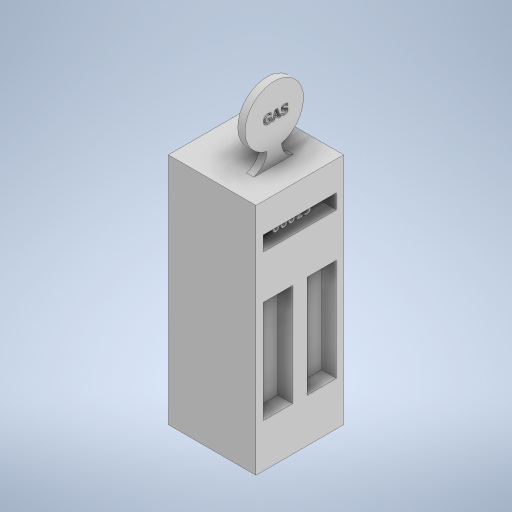
# Autodesk Inventor part: gaspomp
Saved by Autodesk Inventor 2023 (Build 270158000, 158)
## iProperties
Created: 2023-06-06
Part Number: gaspomp
Material: Generic
Document SubType Name: Modeling
Designer: Prestige
Density: 1 g/cm^3
Appearance: Default
Author: Prestige
Autodesk Inventor part; units mm, degrees
ref_plane "YZ Plane" through (0, 0, 0) normal (1, 0, 0) x (0, 1, 0)
ref_plane "XZ Plane" through (0, 0, 0) normal (0, 1, 0) x (-1, 0, 0)
ref_plane "XY Plane" through (0, 0, 0) normal (0, 0, 1) x (1, 0, 0)
sketch "Sketch1" plane through (0, 0, 0) normal (0, 1, 0) x (-1, 0, 0)
  line L0 (0, 0) -> (10, 0)
  line L1 (10, 0) -> (10, -10)
  line L2 (10, -10) -> (0, -10)
  line L3 (0, -10) -> (0, 0)
  dimension "d0" = 10
  dimension "d1" = 10
  constraints: 8 end point, 2 parallel, 1 horizontal, 1 perpendicular
  measures "d0" distance of L0.end L1.end
  measures "d1" distance of L1.end L2.end
extrude "Extrusion1" add sketch "Sketch1" along normal blind 5
sketch "Sketch2" plane through (0, 5, 0) normal (0, 1, 0) x (1, 0, 0)
  line L0 (10, -10) -> (-20, -10)
  line L1 (-20, -10) -> (-20, 20)
  line L2 (-20, 20) -> (10, 20)
  line L3 (10, 20) -> (10, -10)
  line L4 (0, 10) -> (-10, 10) projected
  line L5 (-10, 10) -> (-10, 0) projected
  point P0 (0, 0)
  point P1 (-5, 10)
  point P2 (-10, 5)
  dimension "d4" = 30
  dimension "d5" = 30
  dimension "d6" = 10
  dimension "d7" = 10
  constraints: 8 end point, 2 midpoint, 2 parallel, 1 horizontal, 1 perpendicular
  measures "d4" distance of L0.end L1.end
  measures "d5" distance of L1.end L2.end
  measures "d6" distance from line of point (-5, 10) L2
  measures "d7" distance from line of L1 point (-10, 5)
extrude "Extrusion2" add sketch "Sketch2" along normal blind 80
sketch "Sketch3" plane through (0, 0, 0) normal (1, 0, 0) x (0, 1, 0)
  arc A0 (90.3175, -7.5) -> (90.3175, -2.5) centre (100, -5) ccw
  line L0 (85, 10) -> (85, -20) projected
  line L1 (85, -20) -> (85, 10) projected
  line L2 (85, -2.5) -> (85, -7.5)
  line L3 (5, 10) -> (85, 10) projected
  arc A1 (90.3175, -7.5) -> (85, -14.4535) centre (90.3175, -13.01) ccw
  arc A2 (85, 5) -> (90.3175, -2.5) centre (90.8491, 3.5119) ccw
  point P0 (0, 0)
  point P1 (87.6588, -2.5)
  point P2 (85, 2.0239)
  point P3 (85, -11.5665)
  dimension "d10" = 20
  dimension "d11" = 15
  dimension "d13" = 2.5
  dimension "d14" = 15
  constraints: 6 point on circle, 3 centre point, 3 point on line, 2 end point
  measures "d10" diameter of A0
  measures "d11" distance from line of L0 A0.centre
  measures "d13" vertical distance of A0.centre point (87.659, -2.5)
  measures "d14" distance from line of L3 A0.centre
extrude "Extrusion3" add sketch "Sketch3" along normal mid plane 2.5 contours A1 L0 A2 A0
sketch "Sketch4" plane through (1.25, 0, 0) normal (1, 0, 0) x (0, 0, -1)
  line L0 (1.1377, 101.4111) -> (14.2751, 101.4111) construction
  line L1 (14.2751, 101.4111) -> (14.2751, 95.9848) construction
  line L2 (14.2751, 95.9848) -> (1.1377, 95.9848) construction
  line L3 (1.1377, 95.9848) -> (1.1377, 101.4111) construction
  spline S0 degree 2 poles (3.9999, 98.4748) (3.7997, 98.3933) (3.1595, 98.2376) (2.8481, 98.2376) knots 0 0 0 1 2 2 2
  spline S1 degree 2 poles (2.8481, 98.2376) (2.1289, 98.2376) (1.2761, 99.068) (1.2761, 99.8293) knots 0 0 0 1 2 2 2
  spline S2 degree 2 poles (1.2761, 99.8293) (1.2761, 100.5461) (2.1289, 101.4111) (2.8703, 101.4111) knots 0 0 0 1 2 2 2
  spline S3 degree 2 poles (2.8703, 101.4111) (3.2535, 101.4111) (3.7329, 101.2653) (3.9875, 101.1417) knots 0 0 0 1 2 2 2
  line L4 (3.9875, 101.1417) -> (3.9875, 100.425)
  line L5 (3.9875, 100.425) -> (3.9183, 100.425)
  spline S4 degree 2 poles (3.9183, 100.425) (3.8639, 100.467) (3.6563, 100.6276) (3.5575, 100.682) knots 0 0 0 1 2 2 2
  spline S5 degree 2 poles (3.5575, 100.682) (3.4438, 100.7487) (3.1422, 100.8427) (2.9742, 100.8427) knots 0 0 0 1 2 2 2
  spline S6 degree 2 poles (2.9742, 100.8427) (2.7789, 100.8427) (2.4551, 100.7191) (2.3291, 100.593) knots 0 0 0 1 2 2 2
  spline S7 degree 2 poles (2.3291, 100.593) (2.2079, 100.4694) (2.0671, 100.0913) (2.0671, 99.8416) knots 0 0 0 1 2 2 2
  spline S8 degree 2 poles (2.0671, 99.8416) (2.0671, 99.3078) (2.6034, 98.7986) (3.0656, 98.7986) knots 0 0 0 1 2 2 2
  spline S9 degree 2 poles (3.0656, 98.7986) (3.1076, 98.7986) (3.2164, 98.8036) (3.2584, 98.806) knots 0 0 0 1 2 2 2
  line L6 (3.2584, 98.806) -> (3.2584, 99.4066)
  line L7 (3.2584, 99.4066) -> (2.6677, 99.4066)
  line L8 (2.6677, 99.4066) -> (2.6677, 99.9776)
  line L9 (2.6677, 99.9776) -> (3.9999, 99.9776)
  line L10 (3.9999, 99.9776) -> (3.9999, 98.4748)
  line L11 (4.2495, 98.3018) -> (5.2802, 101.3518)
  line L12 (5.2802, 101.3518) -> (6.1156, 101.3518)
  line L13 (6.1156, 101.3518) -> (7.1463, 98.3018)
  line L14 (7.1463, 98.3018) -> (6.3578, 98.3018)
  line L15 (6.3578, 98.3018) -> (6.1675, 98.9247)
  line L16 (6.1675, 98.9247) -> (5.2085, 98.9247)
  line L17 (5.2085, 98.9247) -> (5.0157, 98.3018)
  line L18 (5.0157, 98.3018) -> (4.2495, 98.3018)
  line L19 (5.9994, 99.4783) -> (5.688, 100.4867)
  line L20 (5.688, 100.4867) -> (5.3741, 99.4783)
  line L21 (5.3741, 99.4783) -> (5.9994, 99.4783)
  spline S10 degree 2 poles (8.392, 98.2474) (8.041, 98.2474) (7.5121, 98.3834) (7.2847, 98.4822) knots 0 0 0 1 2 2 2
  line L22 (7.2847, 98.4822) -> (7.2847, 99.2089)
  line L23 (7.2847, 99.2089) -> (7.3539, 99.2089)
  spline S11 degree 2 poles (7.3539, 99.2089) (7.5838, 99.0137) (8.1349, 98.8036) (8.3945, 98.8036) knots 0 0 0 1 2 2 2
  spline S12 degree 2 poles (8.3945, 98.8036) (8.4612, 98.8036) (8.6762, 98.8332) (8.7405, 98.8629) knots 0 0 0 1 2 2 2
  spline S13 degree 2 poles (8.7405, 98.8629) (8.8196, 98.8975) (8.9308, 99.0235) (8.9308, 99.1249) knots 0 0 0 1 2 2 2
  spline S14 degree 2 poles (8.9308, 99.1249) (8.9308, 99.241) (8.7504, 99.3844) (8.6268, 99.4165) knots 0 0 0 1 2 2 2
  spline S15 degree 2 poles (8.6268, 99.4165) (8.4711, 99.4585) (8.1176, 99.5302) (7.9619, 99.5846) knots 0 0 0 1 2 2 2
  spline S16 degree 2 poles (7.9619, 99.5846) (7.6085, 99.7082) (7.302, 100.1308) (7.302, 100.4472) knots 0 0 0 1 2 2 2
  spline S17 degree 2 poles (7.302, 100.4472) (7.302, 100.8748) (8.0262, 101.4062) (8.5699, 101.4062) knots 0 0 0 1 2 2 2
  spline S18 degree 2 poles (8.5699, 101.4062) (8.8418, 101.4062) (9.3806, 101.295) (9.5932, 101.201) knots 0 0 0 1 2 2 2
  line L24 (9.5932, 101.201) -> (9.5932, 100.504)
  line L25 (9.5932, 100.504) -> (9.5265, 100.504)
  spline S19 degree 2 poles (9.5265, 100.504) (9.3559, 100.6499) (8.8665, 100.8501) (8.6095, 100.8501) knots 0 0 0 1 2 2 2
  spline S20 degree 2 poles (8.6095, 100.8501) (8.5082, 100.8501) (8.35, 100.8204) (8.261, 100.7809) knots 0 0 0 1 2 2 2
  spline S21 degree 2 poles (8.261, 100.7809) (8.1893, 100.7487) (8.0855, 100.6202) (8.0855, 100.5411) knots 0 0 0 1 2 2 2
  spline S22 degree 2 poles (8.0855, 100.5411) (8.0855, 100.4225) (8.2511, 100.2865) (8.4884, 100.2322) knots 0 0 0 1 2 2 2
  spline S23 degree 2 poles (8.4884, 100.2322) (8.6416, 100.1976) (8.9259, 100.1308) (9.089, 100.074) knots 0 0 0 1 2 2 2
  spline S24 degree 2 poles (9.089, 100.074) (9.4054, 99.9578) (9.7143, 99.5722) (9.7143, 99.2559) knots 0 0 0 1 2 2 2
  spline S25 degree 2 poles (9.7143, 99.2559) (9.7143, 98.8011) (9, 98.2474) (8.392, 98.2474) knots 0 0 0 1 2 2 2
  point P0 (0, 0)
  constraints: 2 other
extrude "Extrusion4" cut sketch "Sketch4" against normal blind 2.5
sketch "Sketch5" plane through (10, 5, 10) normal (1, 0, 0) x (0, 0, -1)
  line L0 (2.5, 70) -> (27.5, 70)
  line L1 (27.5, 70) -> (27.5, 65)
  line L2 (27.5, 65) -> (2.5, 65)
  line L3 (2.5, 65) -> (2.5, 70)
  line L4 (17.5, 50) -> (27.5, 50)
  line L5 (27.5, 50) -> (27.5, 15)
  line L6 (27.5, 15) -> (17.5, 15)
  line L7 (17.5, 15) -> (17.5, 50)
  line L8 (2.5, 50) -> (12.5, 50)
  line L9 (12.5, 50) -> (12.5, 15)
  line L10 (12.5, 15) -> (2.5, 15)
  line L11 (2.5, 15) -> (2.5, 50)
  line L12 (0, 80) -> (30, 80) projected
  line L13 (30, 0) -> (30, 80) projected
  point P0 (10, -5)
  dimension "d19" = 10
  dimension "d20" = 5
  dimension "d21" = 25
  dimension "d22" = 2.5
  dimension "d23" = 10
  dimension "d24" = 10
  dimension "d25" = 15
  dimension "d26" = 15
  dimension "d27" = 35
  constraints: 24 end point, 6 parallel, 3 horizontal, 3 perpendicular, 3 point on line
  measures "d19" distance between parallel lines of L12 L0
  measures "d20" distance of L0.end L1.end
  measures "d21" distance of L0.start L0.end
  measures "d22" distance between parallel lines of L13 L1
  measures "d23" distance of L8.start L8.end
  measures "d24" distance of L4.start L4.end
  measures "d25" distance between parallel lines of L2 L8
  measures "d26" distance between parallel lines of L2 L4
  measures "d27" distance of L4.end L5.end
extrude "Extrusion5" cut sketch "Sketch5" against normal blind 5
sketch "Sketch6" plane through (5, 5, 10) normal (1, 0, 0) x (0, 0, -1)
  line L0 (8.0385, 69.3274) -> (32.814, 69.3274) construction
  line L1 (32.814, 69.3274) -> (32.814, 64.0237) construction
  line L2 (32.814, 64.0237) -> (8.0385, 64.0237) construction
  line L3 (8.0385, 64.0237) -> (8.0385, 69.3274) construction
  spline S0 degree 2 poles (10.5496, 67.7381) (10.5496, 67.3426) (10.4236, 66.7494) (10.2827, 66.5492) knots 0 0 0 1 2 2 2
  spline S1 degree 2 poles (10.2827, 66.5492) (10.1443, 66.3515) (9.6969, 66.1488) (9.3756, 66.1488) knots 0 0 0 1 2 2 2
  spline S2 degree 2 poles (9.3756, 66.1488) (9.0518, 66.1488) (8.6069, 66.3515) (8.4661, 66.5542) knots 0 0 0 1 2 2 2
  spline S3 degree 2 poles (8.4661, 66.5542) (8.3252, 66.7544) (8.1991, 67.3426) (8.1991, 67.7381) knots 0 0 0 1 2 2 2
  spline S4 degree 2 poles (8.1991, 67.7381) (8.1991, 68.1434) (8.3252, 68.7169) (8.4685, 68.9245) knots 0 0 0 1 2 2 2
  spline S5 degree 2 poles (8.4685, 68.9245) (8.6119, 69.1271) (9.0642, 69.3249) (9.3756, 69.3249) knots 0 0 0 1 2 2 2
  spline S6 degree 2 poles (9.3756, 69.3249) (9.7043, 69.3249) (10.1443, 69.1173) (10.2852, 68.9121) knots 0 0 0 1 2 2 2
  spline S7 degree 2 poles (10.2852, 68.9121) (10.4236, 68.7119) (10.5496, 68.1212) (10.5496, 67.7381) knots 0 0 0 1 2 2 2
  spline S8 degree 2 poles (9.781, 67.7381) (9.781, 68.3041) (9.5956, 68.7613) (9.3756, 68.7613) knots 0 0 0 1 2 2 2
  spline S9 degree 2 poles (9.3756, 68.7613) (9.1556, 68.7613) (8.9678, 68.3041) (8.9678, 67.7356) knots 0 0 0 1 2 2 2
  spline S10 degree 2 poles (8.9678, 67.7356) (8.9678, 67.177) (9.1556, 66.7124) (9.3756, 66.7124) knots 0 0 0 1 2 2 2
  spline S11 degree 2 poles (9.3756, 66.7124) (9.5931, 66.7124) (9.781, 67.177) (9.781, 67.7381) knots 0 0 0 1 2 2 2
  spline S12 degree 2 poles (13.2215, 67.7381) (13.2215, 67.3426) (13.0954, 66.7494) (12.9545, 66.5492) knots 0 0 0 1 2 2 2
  spline S13 degree 2 poles (12.9545, 66.5492) (12.8161, 66.3515) (12.3688, 66.1488) (12.0475, 66.1488) knots 0 0 0 1 2 2 2
  spline S14 degree 2 poles (12.0475, 66.1488) (11.7237, 66.1488) (11.2788, 66.3515) (11.1379, 66.5542) knots 0 0 0 1 2 2 2
  spline S15 degree 2 poles (11.1379, 66.5542) (10.997, 66.7544) (10.871, 67.3426) (10.871, 67.7381) knots 0 0 0 1 2 2 2
  spline S16 degree 2 poles (10.871, 67.7381) (10.871, 68.1434) (10.997, 68.7169) (11.1404, 68.9245) knots 0 0 0 1 2 2 2
  spline S17 degree 2 poles (11.1404, 68.9245) (11.2837, 69.1271) (11.736, 69.3249) (12.0475, 69.3249) knots 0 0 0 1 2 2 2
  spline S18 degree 2 poles (12.0475, 69.3249) (12.3762, 69.3249) (12.8161, 69.1173) (12.957, 68.9121) knots 0 0 0 1 2 2 2
  spline S19 degree 2 poles (12.957, 68.9121) (13.0954, 68.7119) (13.2215, 68.1212) (13.2215, 67.7381) knots 0 0 0 1 2 2 2
  spline S20 degree 2 poles (12.4528, 67.7381) (12.4528, 68.3041) (12.2674, 68.7613) (12.0475, 68.7613) knots 0 0 0 1 2 2 2
  spline S21 degree 2 poles (12.0475, 68.7613) (11.8275, 68.7613) (11.6396, 68.3041) (11.6396, 67.7356) knots 0 0 0 1 2 2 2
  spline S22 degree 2 poles (11.6396, 67.7356) (11.6396, 67.177) (11.8275, 66.7124) (12.0475, 66.7124) knots 0 0 0 1 2 2 2
  spline S23 degree 2 poles (12.0475, 66.7124) (12.265, 66.7124) (12.4528, 67.177) (12.4528, 67.7381) knots 0 0 0 1 2 2 2
  spline S24 degree 2 poles (15.8933, 67.7381) (15.8933, 67.3426) (15.7673, 66.7494) (15.6264, 66.5492) knots 0 0 0 1 2 2 2
  spline S25 degree 2 poles (15.6264, 66.5492) (15.488, 66.3515) (15.0406, 66.1488) (14.7193, 66.1488) knots 0 0 0 1 2 2 2
  spline S26 degree 2 poles (14.7193, 66.1488) (14.3955, 66.1488) (13.9506, 66.3515) (13.8097, 66.5542) knots 0 0 0 1 2 2 2
  spline S27 degree 2 poles (13.8097, 66.5542) (13.6688, 66.7544) (13.5428, 67.3426) (13.5428, 67.7381) knots 0 0 0 1 2 2 2
  spline S28 degree 2 poles (13.5428, 67.7381) (13.5428, 68.1434) (13.6688, 68.7169) (13.8122, 68.9245) knots 0 0 0 1 2 2 2
  spline S29 degree 2 poles (13.8122, 68.9245) (13.9556, 69.1271) (14.4079, 69.3249) (14.7193, 69.3249) knots 0 0 0 1 2 2 2
  spline S30 degree 2 poles (14.7193, 69.3249) (15.048, 69.3249) (15.488, 69.1173) (15.6289, 68.9121) knots 0 0 0 1 2 2 2
  spline S31 degree 2 poles (15.6289, 68.9121) (15.7673, 68.7119) (15.8933, 68.1212) (15.8933, 67.7381) knots 0 0 0 1 2 2 2
  spline S32 degree 2 poles (15.1246, 67.7381) (15.1246, 68.3041) (14.9393, 68.7613) (14.7193, 68.7613) knots 0 0 0 1 2 2 2
  spline S33 degree 2 poles (14.7193, 68.7613) (14.4993, 68.7613) (14.3115, 68.3041) (14.3115, 67.7356) knots 0 0 0 1 2 2 2
  spline S34 degree 2 poles (14.3115, 67.7356) (14.3115, 67.177) (14.4993, 66.7124) (14.7193, 66.7124) knots 0 0 0 1 2 2 2
  spline S35 degree 2 poles (14.7193, 66.7124) (14.9368, 66.7124) (15.1246, 67.177) (15.1246, 67.7381) knots 0 0 0 1 2 2 2
  line L4 (18.6047, 66.2131) -> (16.3629, 66.2131)
  line L5 (16.3629, 66.2131) -> (16.3629, 66.7099)
  spline S36 degree 2 poles (16.3629, 66.7099) (16.6472, 66.9373) (17.102, 67.3377) (17.2725, 67.5181) knots 0 0 0 1 2 2 2
  spline S37 degree 2 poles (17.2725, 67.5181) (17.4974, 67.7529) (17.6976, 68.1113) (17.6976, 68.2991) knots 0 0 0 1 2 2 2
  spline S38 degree 2 poles (17.6976, 68.2991) (17.6976, 68.5117) (17.443, 68.7391) (17.2156, 68.7391) knots 0 0 0 1 2 2 2
  spline S39 degree 2 poles (17.2156, 68.7391) (17.0995, 68.7391) (16.8919, 68.6823) (16.7856, 68.6378) knots 0 0 0 1 2 2 2
  spline S40 degree 2 poles (16.7856, 68.6378) (16.6818, 68.5908) (16.5335, 68.4919) (16.4964, 68.4672) knots 0 0 0 1 2 2 2
  line L6 (16.4964, 68.4672) -> (16.4371, 68.4672)
  line L7 (16.4371, 68.4672) -> (16.4371, 69.1321)
  spline S41 degree 2 poles (16.4371, 69.1321) (16.5656, 69.1939) (17.1143, 69.3224) (17.3689, 69.3224) knots 0 0 0 1 2 2 2
  spline S42 degree 2 poles (17.3689, 69.3224) (17.9127, 69.3224) (18.4712, 68.838) (18.4712, 68.4005) knots 0 0 0 1 2 2 2
  spline S43 degree 2 poles (18.4712, 68.4005) (18.4712, 68.1311) (18.2167, 67.612) (17.9225, 67.3154) knots 0 0 0 1 2 2 2
  spline S44 degree 2 poles (17.9225, 67.3154) (17.7372, 67.1325) (17.3887, 66.8483) (17.312, 66.789) knots 0 0 0 1 2 2 2
  line L8 (17.312, 66.789) -> (18.6047, 66.789)
  line L9 (18.6047, 66.789) -> (18.6047, 66.2131)
  spline S45 degree 2 poles (21.1999, 67.1375) (21.1999, 66.9126) (21.0343, 66.5443) (20.8737, 66.4158) knots 0 0 0 1 2 2 2
  spline S46 degree 2 poles (20.8737, 66.4158) (20.713, 66.2872) (20.2755, 66.1488) (19.9616, 66.1488) knots 0 0 0 1 2 2 2
  spline S47 degree 2 poles (19.9616, 66.1488) (19.6057, 66.1488) (19.0966, 66.2675) (18.9359, 66.3416) knots 0 0 0 1 2 2 2
  line L10 (18.9359, 66.3416) -> (18.9359, 67.004)
  line L11 (18.9359, 67.004) -> (19.0101, 67.004)
  spline S48 degree 2 poles (19.0101, 67.004) (19.1781, 66.8977) (19.6304, 66.7395) (19.8183, 66.7395) knots 0 0 0 1 2 2 2
  spline S49 degree 2 poles (19.8183, 66.7395) (19.9295, 66.7395) (20.189, 66.7791) (20.278, 66.8434) knots 0 0 0 1 2 2 2
  spline S50 degree 2 poles (20.278, 66.8434) (20.3472, 66.8953) (20.4312, 67.046) (20.4312, 67.182) knots 0 0 0 1 2 2 2
  spline S51 degree 2 poles (20.4312, 67.182) (20.4312, 67.3179) (20.3126, 67.4637) (20.2137, 67.4983) knots 0 0 0 1 2 2 2
  spline S52 degree 2 poles (20.2137, 67.4983) (20.1149, 67.5329) (19.8405, 67.5404) (19.7342, 67.5404) knots 0 0 0 1 2 2 2
  line L12 (19.7342, 67.5404) -> (19.6033, 67.5404)
  line L13 (19.6033, 67.5404) -> (19.6033, 68.0767)
  line L14 (19.6033, 68.0767) -> (19.7244, 68.0767)
  spline S53 degree 2 poles (19.7244, 68.0767) (19.8628, 68.0767) (20.0976, 68.1014) (20.1791, 68.1385) knots 0 0 0 1 2 2 2
  spline S54 degree 2 poles (20.1791, 68.1385) (20.2607, 68.178) (20.3522, 68.3165) (20.3522, 68.4351) knots 0 0 0 1 2 2 2
  spline S55 degree 2 poles (20.3522, 68.4351) (20.3522, 68.529) (20.2656, 68.6452) (20.2039, 68.6773) knots 0 0 0 1 2 2 2
  spline S56 degree 2 poles (20.2039, 68.6773) (20.1297, 68.7144) (19.932, 68.7391) (19.8628, 68.7391) knots 0 0 0 1 2 2 2
  spline S57 degree 2 poles (19.8628, 68.7391) (19.7515, 68.7391) (19.5167, 68.6872) (19.408, 68.6452) knots 0 0 0 1 2 2 2
  spline S58 degree 2 poles (19.408, 68.6452) (19.3215, 68.613) (19.1336, 68.5092) (19.0891, 68.4821) knots 0 0 0 1 2 2 2
  line L15 (19.0891, 68.4821) -> (19.0249, 68.4821)
  line L16 (19.0249, 68.4821) -> (19.0249, 69.1346)
  spline S59 degree 2 poles (19.0249, 69.1346) (19.1831, 69.2013) (19.7169, 69.3274) (19.9962, 69.3274) knots 0 0 0 1 2 2 2
  spline S60 degree 2 poles (19.9962, 69.3274) (20.2681, 69.3274) (20.6685, 69.2334) (20.8094, 69.142) knots 0 0 0 1 2 2 2
  spline S61 degree 2 poles (20.8094, 69.142) (20.9651, 69.0456) (21.1208, 68.749) (21.1208, 68.5636) knots 0 0 0 1 2 2 2
  spline S62 degree 2 poles (21.1208, 68.5636) (21.1208, 68.3016) (20.8193, 67.9111) (20.5721, 67.8543) knots 0 0 0 1 2 2 2
  line L17 (20.5721, 67.8543) -> (20.5721, 67.8246)
  spline S63 degree 2 poles (20.5721, 67.8246) (20.6809, 67.8098) (20.8885, 67.7307) (20.9874, 67.6417) knots 0 0 0 1 2 2 2
  spline S64 degree 2 poles (20.9874, 67.6417) (21.0788, 67.5626) (21.1999, 67.3105) (21.1999, 67.1375) knots 0 0 0 1 2 2 2
  point P0 (10, -5)
  constraints: 2 other
extrude "Extrusion6" add sketch "Sketch6" along normal blind 2.5
body "Solid1"
